Axe 1 (Autodesk Fusion 360 design; units mm, degrees)
Autodesk Fusion 360 part; units mm, degrees
sketch "Sketch1" plane through (0, 0, 0) normal (0, 0, 1) x (1, 0, 0)
  line L0 (-5.7735, 10) -> (-11.547, 0)
  line L1 (-11.547, 0) -> (-5.7735, -10)
  line L2 (-5.7735, -10) -> (5.7735, -10)
  line L3 (5.7735, -10) -> (11.547, 0)
  line L4 (11.547, 0) -> (5.7735, 10)
  line L5 (5.7735, 10) -> (-5.7735, 10)
  circle A0 centre (0, 0) radius 1.75
  dimension "d1" = 20
  dimension "d15" = 3.5
  constraint coincident A0.centre origin
  measures "d1" distance of L2 L5
  measures "d15" diameter of A0
extrude "Extrude1" add sketch "Sketch1" along normal blind 3
sketch "Sketch2" plane through (0, 0, 3) normal (0, 0, 1) x (-1, 0, 0)
  line L0 (-5.7735, -10) -> (5.7735, -10)
  line L1 (5.7735, -10) -> (11.547, 0)
  line L2 (11.547, 0) -> (5.7735, 10)
  line L3 (5.7735, 10) -> (-5.7735, 10)
  line L4 (-5.7735, 10) -> (-11.547, 0)
  line L5 (-11.547, 0) -> (-5.7735, -10)
  circle A0 centre (0, 0) radius 5.9
  circle A1 centre (0, 0) radius 1.75
  dimension "d4" = 11.8
  constraint coincident A0.centre A1.centre
  measures "d4" diameter of A0
extrude "Extrude2" add sketch "Sketch2" along normal blind 16 contours A0
sketch "Sketch4" plane through (0, 0, 19) normal (0, 0, 1) x (-1, 0, 0)
  circle A0 centre (0, 0) radius 4
  line L0 (1.963, -3.4) -> (3.926, 0)
  line L1 (3.926, 0) -> (1.963, 3.4)
  line L2 (1.963, 3.4) -> (-1.963, 3.4)
  line L3 (-1.963, 3.4) -> (-3.926, 0)
  line L4 (-3.926, 0) -> (-1.963, -3.4)
  line L5 (-1.963, -3.4) -> (1.963, -3.4)
  circle A1 centre (0, 0) radius 5.9
  circle A2 centre (0, 0) radius 1.75
  dimension "d16" = 6.8
  constraint coincident A0.centre A1.centre
  measures "d16" distance of L2 L5
extrude "Extrude4" cut sketch "Sketch4" against normal blind 10 contours L0 L1 L2 L3 L4 L5
named bodies: "Axe1"
